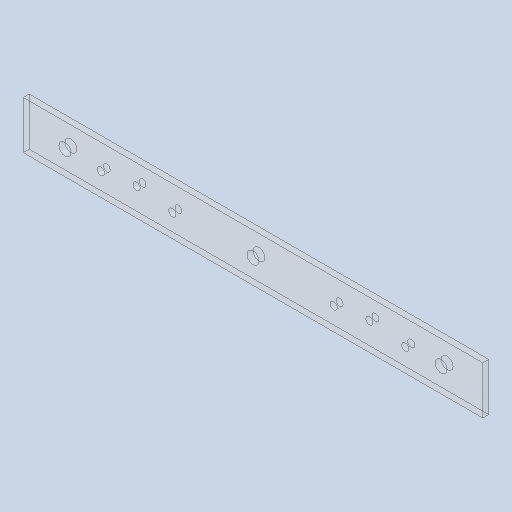
# Autodesk Inventor part: Sup.Acrilico
Saved by Autodesk Inventor 2022 (Build 260153000, 153)
## iProperties
Created: 2018-06-05
Part Number: Sup.Acrilico
Material: Acrílico, claro
Document SubType Name: Modeling
Designer: Cristiano
Density: 1.19 g/cm^3
Appearance: Transparente - Claro
Mass: 228.657 g
Surface Area: 496.128 cm^2
Volume: 300.865 cm^3
Author: Cristiano
Autodesk Inventor part; units mm, degrees
ref_plane "YZ Plane" through (0, 0, 0) normal (1, 0, 0) x (0, 1, 0)
ref_plane "XZ Plane" through (0, 0, 0) normal (0, 1, 0) x (-1, 0, 0)
ref_plane "XY Plane" through (0, 0, 0) normal (0, 0, 1) x (1, 0, 0)
sketch "Boceto1" plane through (0, 0, 0) normal (0, 0, 1) x (1, 0, 0)
  line L0 (0, 0) -> (385, 0)
  line L1 (385, 0) -> (385, 40)
  line L2 (385, 40) -> (0, 40)
  line L3 (0, 40) -> (0, 0)
  line L4 (0, 20) -> (385, 20) construction
  circle A0 centre (35, 20) radius 5
  circle A1 centre (192.5, 20) radius 5
  circle A2 centre (350, 20) radius 5
  dimension "d0" = 40
  dimension "d1" = 385
  dimension "d2" = 10
  dimension "d3" = 10
  dimension "d4" = 10
  dimension "d5" = 35
  dimension "d6" = 35
  constraints: 10 end point, 3 centre point, 3 midpoint, 2 parallel, 2 point on line, 1 horizontal, 1 perpendicular
  measures "d0" distance of L2.end L0.start
  measures "d1" distance of L0.start L0.end
  measures "d2" diameter of A0
  measures "d3" diameter of A1
  measures "d4" diameter of A2
  measures "d5" distance of L4.start A0.centre
  measures "d6" distance from line of L1 A2.centre
extrude "Extrusión1" add sketch "Boceto1" along normal blind 5
sketch "Boceto2" plane through (0, 0, 5) normal (0, 0, 1) x (1, 0, 0)
  circle A0 centre (65, 19) radius 3
  circle A1 centre (95, 23) radius 3
  circle A2 centre (125, 19) radius 3
  circle A3 centre (260, 19) radius 3
  circle A4 centre (290, 23) radius 3
  circle A5 centre (320, 19) radius 3
  line L0 (0, 40) -> (0, 0) projected
  line L1 (385, 0) -> (385, 40) projected
  line L2 (0, 0) -> (385, 0) projected
  dimension "d14" = 6
  dimension "d15" = 6
  dimension "d17" = 6
  dimension "d18" = 30
  dimension "d20" = 60
  dimension "d21" = 30
  dimension "d26" = 4
  dimension "d27" = 4
  dimension "d28" = 65
  dimension "d29" = 65
  dimension "d30" = 19
  dimension "d31" = 19
  dimension "d32" = 60
  constraints: 6 centre point, 3 equal radius, 2 horizontal alignment
  measures "d14" diameter of A0
  measures "d15" diameter of A2
  measures "d17" diameter of A1
  measures "d18" horizontal distance of A0.centre A1.centre
  measures "d20" distance of A3.centre A5.centre
  measures "d21" horizontal distance of A4.centre A5.centre
  measures "d26" vertical distance of A0.centre A1.centre
  measures "d27" vertical distance of A3.centre A4.centre
  measures "d28" distance from line of L0 A0.centre
  measures "d29" distance from line of L1 A5.centre
  measures "d30" distance from line of L2 A0.centre
  measures "d31" distance from line of L2 A5.centre
  measures "d32" distance of A0.centre A2.centre
extrude "Extrusión2" cut sketch "Boceto2" against normal blind 10
